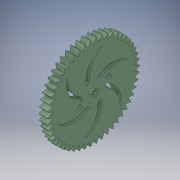
# Autodesk Inventor part: Gear
Saved by Autodesk Inventor 2018 (Build 220112000, 112)
## iProperties
Created: 2018-10-12
Part Number: Gear
Material: Generic
Document SubType Name: Modeling
Designer: 566609
Density: 1 g/cm^3
Appearance: Rubber - Green
Author: 566609
Autodesk Inventor part; units mm, degrees
ref_plane "YZ Plane" through (0, 0, 0) normal (1, 0, 0) x (0, 1, 0)
ref_plane "XZ Plane" through (0, 0, 0) normal (0, 1, 0) x (-1, 0, 0)
ref_plane "XY Plane" through (0, 0, 0) normal (0, 0, 1) x (1, 0, 0)
sketch "Sketch1" plane through (0, 0, 0) normal (1, 0, 0) x (0, 1, 0)
  circle A0 centre (0, 0) radius 32.5
  circle A1 centre (0, 0) radius 2.5
  arc A2 (25.2287, -6.1451) -> (6.4377, 5.2196) centre (9.3901, -11.1162) ccw
  arc A3 (25.2287, -6.1451) -> (7.7879, 3.0884) centre (9.1945, -15.3432) ccw
  line L0 (6.4377, 5.2196) -> (7.7879, 3.0884)
  arc A4 (7.2926, -24.9212) -> (7.7391, -2.9654) centre (-4.9319, -13.6902) ccw
  arc A5 (7.2926, -24.9212) -> (6.5686, -5.2003) centre (-8.6904, -15.6342) ccw
  line L1 (7.7391, -2.9654) -> (6.5686, -5.2003)
  arc A6 (-17.9361, -18.7762) -> (1.3015, -8.185) centre (-14.322, -2.5739) ccw
  arc A7 (-17.9361, -18.7762) -> (-1.2193, -8.2888) centre (-17.8848, -0.291) ccw
  line L2 (1.3015, -8.185) -> (-1.2193, -8.2888)
  arc A8 (-25.2287, 6.1451) -> (-6.4377, -5.2196) centre (-9.3901, 11.1162) ccw
  arc A9 (-25.2287, 6.1451) -> (-7.7879, -3.0884) centre (-9.1945, 15.3432) ccw
  line L3 (-6.4377, -5.2196) -> (-7.7879, -3.0884)
  arc A10 (-7.2926, 24.9212) -> (-7.7391, 2.9654) centre (4.9319, 13.6902) ccw
  arc A11 (-7.2926, 24.9212) -> (-6.5686, 5.2003) centre (8.6904, 15.6342) ccw
  line L4 (-7.7391, 2.9654) -> (-6.5686, 5.2003)
  arc A12 (17.9361, 18.7762) -> (-1.3015, 8.185) centre (14.322, 2.5739) ccw
  arc A13 (17.9361, 18.7762) -> (1.2193, 8.2888) centre (17.8848, 0.291) ccw
  line L5 (-1.3015, 8.185) -> (1.2193, 8.2888)
  circle A14 centre (0, 0) radius 28.5
  dimension "d0" = 65
  dimension "d1" = 30
  dimension "d4" = 360
  dimension "d6" = 4
  constraints: 24 point on circle, 15 centre point, 12 end point, 1 coincident, 49 other
  measures "d0" diameter of A0
  measures "d1" radial gap between concentric circles of A0 A1
  measures "d6" radial gap between concentric circles of A0 A14
extrude "Extrusion1" add sketch "Sketch1" along normal mid plane 6 contours A0 | A14
sketch "Sketch2" plane through (3, 0, 0) normal (1, 0, 0) x (0, 0, -1)
  line L0 (-0.0707, 29.1512) -> (-2.0864, 32.6424)
  line L1 (-2.0864, 32.6424) -> (1.945, 32.6424)
  line L2 (1.945, 32.6424) -> (-0.0707, 29.1512)
  line L3 (2.0213, 32.6465) -> (6.0208, 32.1413)
  line L4 (3.5835, 28.9302) -> (2.0213, 32.6465)
  line L5 (6.0208, 32.1413) -> (3.5835, 28.9302)
  line L6 (6.097, 32.1358) -> (10.0017, 31.1332)
  line L7 (7.1811, 28.2529) -> (6.097, 32.1358)
  line L8 (10.0017, 31.1332) -> (7.1811, 28.2529)
  line L9 (10.0766, 31.1182) -> (13.8249, 29.6342)
  line L10 (10.6655, 27.1301) -> (10.0766, 31.1182)
  line L11 (13.8249, 29.6342) -> (10.6655, 27.1301)
  line L12 (13.8973, 29.6099) -> (17.43, 27.6678)
  line L13 (13.9817, 25.5794) -> (13.8973, 29.6099)
  line L14 (17.43, 27.6678) -> (13.9817, 25.5794)
  line L15 (17.4988, 27.6346) -> (20.7603, 25.2651)
  line L16 (17.0774, 23.6254) -> (17.4988, 27.6346)
  line L17 (20.7603, 25.2651) -> (17.0774, 23.6254)
  line L18 (20.8244, 25.2235) -> (23.7631, 22.4639)
  line L19 (19.9038, 21.2987) -> (20.8244, 25.2235)
  line L20 (23.7631, 22.4639) -> (19.9038, 21.2987)
  line L21 (23.8215, 22.4147) -> (26.3912, 19.3084)
  line L22 (22.4163, 18.6361) -> (23.8215, 22.4147)
  line L23 (26.3912, 19.3084) -> (22.4163, 18.6361)
  line L24 (26.443, 19.2523) -> (28.6031, 15.8485)
  line L25 (24.5753, 15.6797) -> (26.443, 19.2523)
  line L26 (28.6031, 15.8485) -> (24.5753, 15.6797)
  line L27 (28.6474, 15.7863) -> (30.3639, 12.1386)
  line L28 (26.3467, 12.4759) -> (28.6474, 15.7863)
  line L29 (30.3639, 12.1386) -> (26.3467, 12.4759)
  line L30 (30.4001, 12.0713) -> (31.6458, 8.2373)
  line L31 (27.7026, 9.0755) -> (30.4001, 12.0713)
  line L32 (31.6458, 8.2373) -> (27.7026, 9.0755)
  line L33 (31.6733, 8.166) -> (32.4287, 4.2061)
  line L34 (28.6216, 5.5318) -> (31.6733, 8.166)
  line L35 (32.4287, 4.2061) -> (28.6216, 5.5318)
  line L36 (32.447, 4.1319) -> (32.7002, 0.1085)
  line L37 (29.0892, 1.901) -> (32.447, 4.1319)
  line L38 (32.7002, 0.1085) -> (29.0892, 1.901)
  line L39 (32.709, 0.0326) -> (32.4559, -3.9908)
  line L40 (29.0981, -1.7599) -> (32.709, 0.0326)
  line L41 (32.4559, -3.9908) -> (29.0981, -1.7599)
  line L42 (32.4552, -4.0672) -> (31.6998, -8.0271)
  line L43 (28.6481, -5.3929) -> (32.4552, -4.0672)
  line L44 (31.6998, -8.0271) -> (28.6481, -5.3929)
  line L45 (31.6895, -8.1028) -> (30.4438, -11.9369)
  line L46 (27.7463, -8.941) -> (31.6895, -8.1028)
  line L47 (30.4438, -11.9369) -> (27.7463, -8.941)
  line L48 (30.4241, -12.0107) -> (28.7076, -15.6583)
  line L49 (26.4069, -12.348) -> (30.4241, -12.0107)
  line L50 (28.7076, -15.6583) -> (26.4069, -12.348)
  line L51 (28.6789, -15.7291) -> (26.5188, -19.1329)
  line L52 (24.651, -15.5603) -> (28.6789, -15.7291)
  line L53 (26.5188, -19.1329) -> (24.651, -15.5603)
  line L54 (26.4813, -19.1995) -> (23.9117, -22.3057)
  line L55 (22.5064, -18.5272) -> (26.4813, -19.1995)
  line L56 (23.9117, -22.3057) -> (22.5064, -18.5272)
  line L57 (23.8662, -22.3671) -> (20.9275, -25.1267)
  line L58 (20.0069, -21.2019) -> (23.8662, -22.3671)
  line L59 (20.9275, -25.1267) -> (20.0069, -21.2019)
  line L60 (20.8747, -25.1819) -> (17.6132, -27.5515)
  line L61 (17.1918, -23.5422) -> (20.8747, -25.1819)
  line L62 (17.6132, -27.5515) -> (17.1918, -23.5422)
  line L63 (17.5539, -27.5997) -> (14.0212, -29.5418)
  line L64 (14.1056, -25.5113) -> (17.5539, -27.5997)
  line L65 (14.0212, -29.5418) -> (14.1056, -25.5113)
  line L66 (13.9564, -29.5821) -> (10.2081, -31.0662)
  line L67 (10.797, -27.0781) -> (13.9564, -29.5821)
  line L68 (10.2081, -31.0662) -> (10.797, -27.0781)
  line L69 (10.1387, -31.0981) -> (6.234, -32.1006)
  line L70 (7.3181, -28.2178) -> (10.1387, -31.0981)
  line L71 (6.234, -32.1006) -> (7.3181, -28.2178)
  line L72 (6.1611, -32.1236) -> (2.1615, -32.6288)
  line L73 (3.7238, -28.9125) -> (6.1611, -32.1236)
  line L74 (2.1615, -32.6288) -> (3.7238, -28.9125)
  line L75 (2.0864, -32.6424) -> (-1.945, -32.6424)
  line L76 (0.0707, -29.1512) -> (2.0864, -32.6424)
  line L77 (-1.945, -32.6424) -> (0.0707, -29.1512)
  line L78 (-2.0213, -32.6465) -> (-6.0208, -32.1413)
  line L79 (-3.5835, -28.9302) -> (-2.0213, -32.6465)
  line L80 (-6.0208, -32.1413) -> (-3.5835, -28.9302)
  line L81 (-6.097, -32.1358) -> (-10.0017, -31.1332)
  line L82 (-7.1811, -28.2529) -> (-6.097, -32.1358)
  line L83 (-10.0017, -31.1332) -> (-7.1811, -28.2529)
  line L84 (-10.0766, -31.1182) -> (-13.8249, -29.6342)
  line L85 (-10.6655, -27.1301) -> (-10.0766, -31.1182)
  line L86 (-13.8249, -29.6342) -> (-10.6655, -27.1301)
  line L87 (-13.8973, -29.6099) -> (-17.43, -27.6678)
  line L88 (-13.9817, -25.5794) -> (-13.8973, -29.6099)
  line L89 (-17.43, -27.6678) -> (-13.9817, -25.5794)
  line L90 (-17.4988, -27.6346) -> (-20.7603, -25.2651)
  line L91 (-17.0774, -23.6254) -> (-17.4988, -27.6346)
  line L92 (-20.7603, -25.2651) -> (-17.0774, -23.6254)
  line L93 (-20.8244, -25.2235) -> (-23.7631, -22.4639)
  line L94 (-19.9038, -21.2987) -> (-20.8244, -25.2235)
  line L95 (-23.7631, -22.4639) -> (-19.9038, -21.2987)
  line L96 (-23.8215, -22.4147) -> (-26.3912, -19.3084)
  line L97 (-22.4163, -18.6361) -> (-23.8215, -22.4147)
  line L98 (-26.3912, -19.3084) -> (-22.4163, -18.6361)
  line L99 (-26.443, -19.2523) -> (-28.6031, -15.8485)
  line L100 (-24.5753, -15.6797) -> (-26.443, -19.2523)
  line L101 (-28.6031, -15.8485) -> (-24.5753, -15.6797)
  line L102 (-28.6474, -15.7863) -> (-30.3639, -12.1386)
  line L103 (-26.3467, -12.4759) -> (-28.6474, -15.7863)
  line L104 (-30.3639, -12.1386) -> (-26.3467, -12.4759)
  line L105 (-30.4001, -12.0713) -> (-31.6458, -8.2373)
  line L106 (-27.7026, -9.0755) -> (-30.4001, -12.0713)
  line L107 (-31.6458, -8.2373) -> (-27.7026, -9.0755)
  line L108 (-31.6733, -8.166) -> (-32.4287, -4.2061)
  line L109 (-28.6216, -5.5318) -> (-31.6733, -8.166)
  line L110 (-32.4287, -4.2061) -> (-28.6216, -5.5318)
  line L111 (-32.447, -4.1319) -> (-32.7002, -0.1085)
  line L112 (-29.0892, -1.901) -> (-32.447, -4.1319)
  line L113 (-32.7002, -0.1085) -> (-29.0892, -1.901)
  line L114 (-32.709, -0.0326) -> (-32.4559, 3.9908)
  line L115 (-29.0981, 1.7599) -> (-32.709, -0.0326)
  line L116 (-32.4559, 3.9908) -> (-29.0981, 1.7599)
  line L117 (-32.4552, 4.0672) -> (-31.6998, 8.0271)
  line L118 (-28.6481, 5.3929) -> (-32.4552, 4.0672)
  line L119 (-31.6998, 8.0271) -> (-28.6481, 5.3929)
  line L120 (-31.6895, 8.1028) -> (-30.4438, 11.9369)
  line L121 (-27.7463, 8.941) -> (-31.6895, 8.1028)
  line L122 (-30.4438, 11.9369) -> (-27.7463, 8.941)
  line L123 (-30.4241, 12.0107) -> (-28.7076, 15.6583)
  line L124 (-26.4069, 12.348) -> (-30.4241, 12.0107)
  line L125 (-28.7076, 15.6583) -> (-26.4069, 12.348)
  line L126 (-28.6789, 15.7291) -> (-26.5188, 19.1329)
  line L127 (-24.651, 15.5603) -> (-28.6789, 15.7291)
  line L128 (-26.5188, 19.1329) -> (-24.651, 15.5603)
  line L129 (-26.4813, 19.1995) -> (-23.9117, 22.3057)
  line L130 (-22.5064, 18.5272) -> (-26.4813, 19.1995)
  line L131 (-23.9117, 22.3057) -> (-22.5064, 18.5272)
  line L132 (-23.8662, 22.3671) -> (-20.9275, 25.1267)
  line L133 (-20.0069, 21.2019) -> (-23.8662, 22.3671)
  line L134 (-20.9275, 25.1267) -> (-20.0069, 21.2019)
  line L135 (-20.8747, 25.1819) -> (-17.6132, 27.5515)
  line L136 (-17.1918, 23.5422) -> (-20.8747, 25.1819)
  line L137 (-17.6132, 27.5515) -> (-17.1918, 23.5422)
  line L138 (-17.5539, 27.5997) -> (-14.0212, 29.5418)
  line L139 (-14.1056, 25.5113) -> (-17.5539, 27.5997)
  line L140 (-14.0212, 29.5418) -> (-14.1056, 25.5113)
  line L141 (-13.9564, 29.5821) -> (-10.2081, 31.0662)
  line L142 (-10.797, 27.0781) -> (-13.9564, 29.5821)
  line L143 (-10.2081, 31.0662) -> (-10.797, 27.0781)
  line L144 (-10.1387, 31.0981) -> (-6.234, 32.1006)
  line L145 (-7.3181, 28.2178) -> (-10.1387, 31.0981)
  line L146 (-6.234, 32.1006) -> (-7.3181, 28.2178)
  line L147 (-6.1611, 32.1236) -> (-2.1615, 32.6288)
  line L148 (-3.7238, 28.9125) -> (-6.1611, 32.1236)
  line L149 (-2.1615, 32.6288) -> (-3.7238, 28.9125)
  point P0 (0, 0)
  point P1 (34.8848, 34.0844)
  dimension "d11" = 360
  constraints: 300 end point, 302 other
sketch "Sketch3" plane through (3, 0, 0) normal (1, 0, 0) x (0, 0, -1)
  circle A0 centre (10.7192, 4.6104) radius 1.4478
  circle A1 centre (-10.1103, -4.3483) radius 1.4478
  point P0 (0, 0)
  dimension "d15" = 2.8956
  dimension "d16" = 2.8956
  constraints: 2 centre point
  measures "d15" diameter of A0
  measures "d16" diameter of A1
sketch "Sketch4" plane through (3, 0, 0) normal (1, 0, 0) x (0, 0, -1)
  circle A0 centre (0, 0) radius 2.5
  constraints: 1 centre point, 1 coincident
extrude "Extrusion5" cut sketch "Sketch2" against normal through all
extrude "Extrusion6" cut sketch "Sketch3" against normal through all
sketch "Sketch6" plane through (-3, 0, 0) normal (-1, 0, 0) x (0, 0, 1)
  line L0 (0.3556, 1.4986) -> (-0.3556, 1.4986)
  line L1 (-1.4986, 0.3556) -> (-1.4986, -0.3556)
  line L2 (-0.3556, -1.4986) -> (0.3556, -1.4986)
  line L3 (1.4986, -0.3556) -> (1.4986, 0.3556)
  arc A0 (-0.3556, 1.4986) -> (-1.4986, 0.3556) centre (-0.3556, 0.3556) ccw
  arc A1 (1.4986, 0.3556) -> (0.3556, 1.4986) centre (0.3556, 0.3556) ccw
  arc A2 (0.3556, -1.4986) -> (1.4986, -0.3556) centre (0.3556, -0.3556) ccw
  arc A3 (-1.4986, -0.3556) -> (-0.3556, -1.4986) centre (-0.3556, -0.3556) ccw
  line L4 (-0.3556, 2.5651) -> (0.3556, 2.5651)
  arc A4 (2.5651, 0.3556) -> (0.3556, 2.5651) centre (0.3556, 0.3556) ccw
  line L5 (2.5651, 0.3556) -> (2.5651, -0.3556)
  arc A5 (0.3556, -2.5651) -> (2.5651, -0.3556) centre (0.3556, -0.3556) ccw
  line L6 (0.3556, -2.5651) -> (-0.3556, -2.5651)
  arc A6 (-2.5651, -0.3556) -> (-0.3556, -2.5651) centre (-0.3556, -0.3556) ccw
  line L7 (-2.5651, -0.3556) -> (-2.5651, 0.3556)
  arc A7 (-0.3556, 2.5651) -> (-2.5651, 0.3556) centre (-0.3556, 0.3556) ccw
  point P0 (0, 0)
  point P1 (-1.4986, -1.4986)
  point P2 (-1.4986, 1.4986)
  point P3 (1.4986, -1.4986)
  dimension "d28" = 2.9972
  dimension "d29" = 2.9972
  dimension "d30" = 1.143
  constraints: 16 end point, 16 point on circle, 8 centre point, 8 tangent, 6 point on line, 4 parallel, 3 equal radius, 2 perpendicular, 1 horizontal, 7 other
  measures "d28" distance of point (1.499, -1.499) point (-1.499, -1.499)
  measures "d29" distance of point (-1.499, -1.499) point (-1.499, 1.499)
  measures "d30" radius of A0
extrude "Extrusion7" add sketch "Sketch6" against normal blind 7 separate body
body "Solid1"
body "Solid2"
